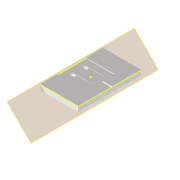
# Autodesk Inventor part: 00_lightsheetchip
Saved by Autodesk Inventor 2022 (Build 260153000, 153)
## iProperties
Created: 2022-01-20
Part Number: 00_lightsheetchip
Material: Generisch
Document SubType Name: Modeling
Designer: diederichbenedict
Density: 1 g/cm^3
Appearance: Vorgabe
Author: diederichbenedict
Autodesk Inventor part; units mm, degrees
ref_plane "YZ Plane" through (0, 0, 0) normal (1, 0, 0) x (0, 1, 0)
ref_plane "XZ Plane" through (0, 0, 0) normal (0, 1, 0) x (-1, 0, 0)
ref_plane "XY Plane" through (0, 0, 0) normal (0, 0, 1) x (1, 0, 0)
sketch "Skizze1" plane through (0, 0, 0) normal (0, 1, 0) x (-1, 0, 0)
  line L0 (-12, -20) -> (12, -20)
  line L1 (12, -20) -> (12, 20)
  line L2 (12, 20) -> (-12, 20)
  line L3 (-12, 20) -> (-12, -20)
  line L4 (-12, -20) -> (12, 20) construction
  line L5 (12, -20) -> (-12, 20) construction
  point P0 (0, 0)
  dimension "d0" = 24
  dimension "d1" = 40
  constraints: 12 end point, 2 midpoint, 2 parallel, 1 horizontal, 1 perpendicular
  measures "d0" distance of L2.end L1.end
  measures "d1" distance of L1.end L0.end
extrude "Extrusion1" add sketch "Skizze1" along normal blind 3
sketch "Skizze2" plane through (0, 3, 0) normal (0, 1, 0) x (1, 0, 0)
  line L0 (-12, 20) -> (-12, -20) projected
  line L1 (-12, -20) -> (12, -20) projected
  line L2 (12, -20) -> (12, 20) projected
  line L3 (12, 20) -> (-12, 20) projected
  point P0 (0, 0)
sketch "Skizze3" plane through (0, 3, 0) normal (0, 1, 0) x (1, 0, 0)
  line L0 (-12, 20) -> (-12, -20) projected
  line L1 (-12, -20) -> (12, -20) projected
  line L2 (12, -20) -> (12, 20) projected
  line L3 (12, 20) -> (-12, 20) projected
  line L4 (-9, -5) -> (6, -5)
  line L5 (6, -5) -> (6, -3)
  line L6 (6, -3) -> (-9, -3)
  line L7 (-9, -3) -> (-9, -5)
  line L8 (6, -3) -> (4, -3)
  line L9 (4, -3) -> (4, 3)
  line L10 (4, 3) -> (6, 3)
  line L11 (6, 3) -> (6, -3)
  line L12 (6, 3) -> (-9, 3)
  line L13 (-9, 3) -> (-9, 5)
  line L14 (-9, 5) -> (6, 5)
  line L15 (6, 5) -> (6, 3)
  point P0 (0, 0)
  point P1 (4, 3)
  point P2 (4, -3)
  dimension "d5" = 2
  dimension "d6" = 2
  dimension "d7" = 6
  dimension "d8" = 2
  dimension "d9" = 3
  dimension "d15" = 18
  dimension "d16" = 3
  dimension "d17" = 3
  constraints: 24 end point, 6 parallel, 3 horizontal, 3 perpendicular
  measures "d5" distance of L5.end L4.end
  measures "d6" distance of L9.end L10.end
  measures "d7" distance of L8.end L9.end
  measures "d8" distance of L12.end L13.end
  measures "d9" distance from line of point (0, 0) L6
  measures "d15" distance between parallel lines of L0 L11
  measures "d16" distance between parallel lines of L0 L7
  measures "d17" distance between parallel lines of L0 L13
extrude "Extrusion2" cut sketch "Skizze3" against normal blind 0.2 contours L7 L6 L5 L4 | L6 L9 L10 L11 | L10 L12 L13 L14 L15
ref_plane "Arbeitsebene1" through (-12, 3, 0) normal (0.7071068, 0.7071068, 0) x (0, 0, -1)
sketch "Skizze5" plane through (-12, 3, 0) normal (0.7071068, 0.7071068, 0) x (0, 0, -1)
  line L0 (5, -12.8693) -> (-5, -12.8693) projected
  line L1 (5, -2.2627) -> (5, -12.8693) projected
  line L2 (3, -2.2627) -> (5, -2.2627) projected
  line L3 (3, -11.4551) -> (3, -2.2627) projected
  line L4 (-3, -11.4551) -> (3, -11.4551) projected
  line L5 (-3, -2.2627) -> (-3, -11.4551) projected
  line L6 (-5, -2.2627) -> (-3, -2.2627) projected
  line L7 (-5, -12.8693) -> (-5, -2.2627) projected
  circle A0 centre (4, -3.5) radius 1.1
  circle A1 centre (-4, -3.5) radius 1.1
  point P0 (0, -10.6066)
  dimension "d18" = 2.2
  dimension "d19" = 2.2
  constraints: 2 centre point
  measures "d18" diameter of A0
  measures "d19" diameter of A1
extrude "Extrusion3" cut sketch "Skizze5" against normal up to surface contours A0 L3 L1 | L1 A0 | A1 L7 | L7 A1 L5 | A0 L3 | L5 A1 surface through (-1.5, 2.8, 0) normal (0, -1, 0)
sketch "Skizze6" plane through (-9.5251, 0.5251, -4) normal (0.7071068, 0.7071068, 0) x (0.7071068, -0.7071068, 0)
  arc A0 (0.4583, -1) -> (0.4583, 1) centre (0, 0) ccw projected
  arc A1 (0.7427, -7.1885) -> (0.7427, -8.8115) centre (0, -8) ccw projected
  arc A2 (0.7427, 0.8115) -> (0.7427, -0.8115) centre (0, 0) ccw projected
  line L0 (0.7427, 0.8115) -> (0.7427, -0.8115) projected
  line L1 (0.7427, -7.1885) -> (0.7427, -8.8115) projected
  point P0 (7.1066, -4)
  point P1 (0.7427, -0.8115)
  point P2 (0.4583, -1)
extrude "Extrusion4" cut sketch "Skizze6" against normal blind 10 contours A2 A0 L0 | L1 A1
sketch "Skizze7" plane through (0, 3, 0) normal (0, 1, 0) x (1, 0, 0)
  line L0 (6, -1.6) -> (12, -1.6)
  line L1 (12, -1.6) -> (12, 1.6)
  line L2 (12, 1.6) -> (6, 1.6)
  line L3 (6, 1.6) -> (6, -1.6)
  line L4 (6, -1.6) -> (12, 1.6) construction
  line L5 (12, -1.6) -> (6, 1.6) construction
  line L6 (6, 5) -> (6, -5) projected
  line L7 (12, -20) -> (12, 20) projected
  point P0 (0, 0)
  point P1 (9, 0)
  point P2 (6, 0)
  point P3 (12, 0)
  dimension "d25" = 3.2
  constraints: 12 end point, 6 midpoint, 2 parallel, 1 horizontal, 1 perpendicular
  measures "d25" distance of L1.end L0.end
extrude "Extrusion5" cut sketch "Skizze7" against normal blind 0.4
fillet "Rundung1" radius 2 4 edges at (6, 2.9, -5) (4, 2.9, -3) (4, 2.9, 3) (6, 2.9, 5)
sketch "Skizze8" plane through (0, 3, 0) normal (0, 1, 0) x (1, 0, 0)
  arc A0 (2, -3) -> (4, -1) centre (2, -1) ccw projected
  line L0 (4, -1) -> (4, 1) projected
  arc A1 (4, 1) -> (2, 3) centre (2, 1) ccw projected
  line L1 (2, 3) -> (-9, 3) projected
  line L2 (-9, 3) -> (-9, 5) projected
  line L3 (-9, 5) -> (4, 5) projected
  arc A2 (6, 3) -> (4, 5) centre (4, 3) ccw projected
  line L4 (6, 3) -> (6, 1.6) projected
  line L5 (6, 1.6) -> (12, 1.6) projected
  line L6 (12, -1.6) -> (6, -1.6) projected
  line L7 (6, -1.6) -> (6, -3) projected
  arc A3 (4, -5) -> (6, -3) centre (4, -3) ccw projected
  line L8 (4, -5) -> (-9, -5) projected
  line L9 (-9, -5) -> (-9, -3) projected
  line L10 (-9, -3) -> (2, -3) projected
  line L11 (-12, 20) -> (-12, -20) projected
  line L12 (-12, -20) -> (12, -20) projected
  line L13 (12, -20) -> (12, -1.6) projected
  line L14 (12, 20) -> (-12, 20) projected
  line L15 (-12, -9.15) -> (6, -9.15)
  line L16 (6, -9.15) -> (6, 9.15)
  line L17 (6, 9.15) -> (-12, 9.15)
  line L18 (-12, 9.15) -> (-12, -9.15)
  line L19 (-12, -9.15) -> (6, 9.15) construction
  line L20 (6, -9.15) -> (-12, 9.15) construction
  line L21 (12, 1.6) -> (12, 20) projected
  point P0 (0, 0)
  point P1 (-3, 0)
  point P2 (-12, 0)
  point P3 (6, -3)
  point P4 (6, 3)
  dimension "d29" = 18
  dimension "d30" = 18.3
  constraints: 12 end point, 4 midpoint, 2 parallel, 1 horizontal, 1 perpendicular
  measures "d29" distance of L17.end L16.end
  measures "d30" distance of L16.end L15.end
extrude "Extrusion6" add sketch "Skizze8" along normal blind 0.5 contours L7 L6 L13 L12 L11 L15 L16 | L4 L16 L17 L11 L14 L21 L5
